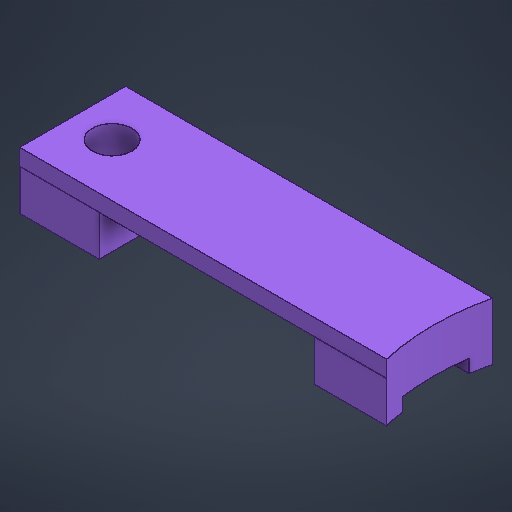
# Autodesk Inventor part: measuring_support1
Saved by Autodesk Inventor 2026.1 (Build 301233000, 233)
## iProperties
Created: 2026-01-06
Part Number: measuring_support1
Material: Generic
Document SubType Name: Modeling
Designer: emanuel
Density: 1 g/cm^3
Appearance: Violet
Author: emanuel
Autodesk Inventor part; units mm, degrees
ref_plane "YZ Plane" through (0, 0, 0) normal (1, 0, 0) x (0, 1, 0)
ref_plane "XZ Plane" through (0, 0, 0) normal (0, 1, 0) x (-1, 0, 0)
ref_plane "XY Plane" through (0, 0, 0) normal (0, 0, 1) x (1, 0, 0)
sketch "Sketch1" plane through (0, 0, 0) normal (0, 1, 0) x (-1, 0, 0)
  circle A0 centre (0, 0) radius 39.95
  circle A1 centre (0, 0) radius 35.05
  line L0 (0, 0) -> (0, -5.05)
  line L1 (0, -5.05) -> (60, -5.05)
  line L2 (60, -5.05) -> (60, 5.05)
  line L3 (60, 5.05) -> (0, 5.05)
  line L4 (0, 5.05) -> (0, -5.05)
  line L5 (0, -5.05) -> (60, -5.05)
  line L6 (60, -5.05) -> (60, -8.05)
  line L7 (60, -8.05) -> (0, -8.05)
  line L8 (0, -8.05) -> (0, -5.05)
  line L9 (0, 5.05) -> (60, 5.05)
  line L10 (60, 5.05) -> (60, 8.05)
  line L11 (60, 8.05) -> (0, 8.05)
  line L12 (0, 8.05) -> (0, 5.05)
  line L13 (39.95, 0) -> (44.95, 0)
  line L14 (44.95, 0) -> (44.95, -8.05)
  line L15 (44.95, 0) -> (44.95, 8.05)
  point P0 (34.113, 8.05)
  point P1 (34.113, -8.05)
  point P2 (44.95, -5.05)
  point P3 (34.6843, -5.05)
  point P4 (34.6843, 5.05)
  point P5 (44.95, 5.05)
  point P6 (39.6295, 5.05)
  point P7 (39.6295, -5.05)
  dimension "d0" = 79.9
  dimension "d1" = 70.1
  dimension "d2" = 5.05
  dimension "d3" = 60
  dimension "d4" = 10.1
  dimension "d5" = 60
  dimension "d6" = 3
  dimension "d7" = 60
  dimension "d8" = 3
  dimension "d9" = 5
  constraints: 32 end point, 6 parallel, 4 horizontal, 4 perpendicular, 3 point on line, 2 coincident, 1 centre point, 1 vertical, 3 other
  measures "d1" diameter of A1
  measures "d2" distance of L0.start L0.end
  measures "d3" distance of L3.end L2.end
  measures "d4" distance of L2.end L1.end
  measures "d5" distance of L6.end L7.end
  measures "d6" distance of L5.end L6.end
  measures "d7" distance of L11.end L10.end
  measures "d8" distance of L10.end L9.end
  measures "d9" distance of L13.start L13.end
extrude "Extrusion1" add sketch "Sketch1" along normal blind 4.2 contours A0 L1 A1 L3 | L13 L14 L1 A0 | A0 L3 L15 L13 | L3 A1 L11 A0 | A0 L11 L15 L3 | L1 L14 L7 A0 | A0 L7 A1 L1
extrude "Extrusion2" add sketch "Sketch1" against normal blind 2 contours L3 A1 L11 A0 | A0 L11 L15 L3 | L1 L14 L7 A0 | A0 L7 A1 L1
extrude "Extrusion3" cut sketch "Sketch1" along normal blind 1 contours L13 L14 L1 A0 | A0 L3 L15 L13
sketch "Sketch2" plane through (0, 4.2, 0) normal (0, 1, 0) x (1, 0, 0)
  line L0 (-44.95, 8.05) -> (-44.95, -8.05) projected
  line L1 (-44.95, 0) -> (-83.7, 0)
  circle A0 centre (-83.7, 0) radius 3
  line L2 (-83.7, 0) -> (-89.7, 0)
  line L3 (-89.7, 0) -> (-89.7, -8)
  line L4 (-89.7, -8) -> (-83.7, -8)
  line L5 (-83.7, -8) -> (-83.7, 0)
  line L6 (-89.7, -8) -> (-44.95, -8)
  line L7 (-44.95, -8) -> (-44.95, 8.05)
  line L8 (-44.95, 8.05) -> (-89.7, 8.05)
  line L9 (-89.7, 8.05) -> (-89.7, -8)
  arc A1 (-34.113, 8.05) -> (-34.113, -8.05) centre (0, 0) ccw projected
  line L10 (-44.95, -8) -> (-34.113, -8)
  line L11 (-34.113, -8) -> (-34.113, 8.05)
  line L12 (-34.113, 8.05) -> (-44.95, 8.05)
  line L13 (-44.95, 8.05) -> (-44.95, -8)
  arc A2 (-34.113, 8.05) -> (-34.113, -8) centre (-0.1059, 0.025) ccw
  point P0 (-34.1248, -8)
  dimension "d16" = 38.75
  dimension "d17" = 6
  dimension "d18" = 6
  dimension "d19" = 8
  constraints: 26 end point, 6 parallel, 4 horizontal, 3 perpendicular, 2 centre point, 2 point on circle, 1 coincident, 1 midpoint, 1 tangent
  measures "d16" distance of L1.start L1.end
  measures "d17" diameter of A0
  measures "d18" distance of L4.end L3.end
  measures "d19" distance of L3.end L2.end
extrude "Extrusion4" add sketch "Sketch2" along normal blind 2.5 contours L12 A1 L10 L0 | L0 L1 A0 L2 L9 L8 | L0 L6 L5 A0 L1 | L2 A0 L5 L4 L3
sketch "Sketch3" plane through (0, 4.2, 0) normal (0, -1, 0) x (1, 0, 0)
  line L0 (-34.113, -8.05) -> (-89.7, -8.05) projected
  line L1 (-89.7, -8.05) -> (-77.7, -8.05)
  line L2 (-77.7, -8.05) -> (-77.7, 7.95)
  line L3 (-77.7, 7.95) -> (-89.7, 7.95)
  line L4 (-89.7, 7.95) -> (-89.7, -8.05)
  circle A0 centre (-83.7, 0) radius 3 projected
  circle A1 centre (-83.7, 0) radius 3
  point P0 (0, 0)
  dimension "d22" = 12
  dimension "d25" = 16
  constraints: 8 end point, 2 parallel, 1 centre point, 1 coincident, 1 horizontal, 1 perpendicular
  measures "d22" distance of L3.end L2.end
  measures "d25" distance of L1.end L2.end
extrude "Extrusion5" add sketch "Sketch3" along normal blind 6.2
body "Solid1"
